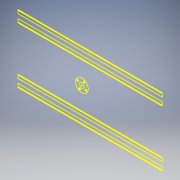
# Autodesk Inventor part: ZNutHolder
Saved by Autodesk Inventor 2019 (Build 230136000, 136)
## iProperties
Created: 2019-05-13
Part Number: ZNutHolder
Material: Generic
Document SubType Name: Modeling
Designer: Alex Jones
Density: 1 g/cm^3
Appearance: Default
Author: Alex Jones
Autodesk Inventor part; units mm, degrees
ref_plane "YZ Plane" through (0, 0, 0) normal (1, 0, 0) x (0, 1, 0)
ref_plane "XZ Plane" through (0, 0, 0) normal (0, 1, 0) x (-1, 0, 0)
ref_plane "XY Plane" through (0, 0, 0) normal (0, 0, 1) x (1, 0, 0)
sketch "Sketch1" plane through (0, 0, 0) normal (0, 0, 1) x (1, 0, 0)
  circle A0 centre (-131.3, 44.85) radius 1.5 projected
  circle A1 centre (-147.3, 44.85) radius 1.5 projected
  circle A2 centre (-139.3, 52.85) radius 1.5 projected
  circle A3 centre (-139.3, 36.85) radius 1.5 projected
  circle A4 centre (-139.3, 44.85) radius 4 projected
  circle A5 centre (-139.3, 44.85) radius 11 projected
  line L0 (-250, 102.05) -> (0, 102.05) projected
  line L1 (-250, 96.9) -> (-250, 102.05) projected
  line L2 (0, 96.9) -> (-250, 96.9) projected
  line L3 (0, 96.9) -> (0, 102.05) projected
  line L4 (0, 103.3) -> (-250, 103.3) projected
  line L5 (0, 84.55) -> (-250, 84.55) projected
  line L6 (0, 84.55) -> (0, 89.7) projected
  line L7 (0, 89.7) -> (-250, 89.7) projected
  line L8 (-250, 84.55) -> (-250, 89.7) projected
  line L9 (-250, 83.3) -> (0, 83.3) projected
  line L10 (-250, 5.15) -> (0, 5.15) projected
  line L11 (-250, 0) -> (-250, 5.15) projected
  line L12 (0, 0) -> (-250, 0) projected
  line L13 (0, 0) -> (0, 5.15) projected
  line L14 (0, -12.35) -> (-250, -12.35) projected
  line L15 (0, -12.35) -> (0, -7.2) projected
  line L16 (0, -7.2) -> (-250, -7.2) projected
  line L17 (-250, -12.35) -> (-250, -7.2) projected
  line L18 (-250, -13.6) -> (0, -13.6) projected
  line L19 (0, 6.4) -> (-250, 6.4) projected
  line L20 (-128.3, 103.3) -> (-150.3, 103.3)
  line L21 (-150.3, 103.3) -> (-150.3, -13.6)
  line L22 (-150.3, -13.6) -> (-128.3, -13.6)
  line L23 (-128.3, -13.6) -> (-128.3, 103.3)
  circle A6 centre (-139.3, 44.85) radius 5.5902
  constraints: 8 end point, 2 parallel, 2 point on line, 2 tangent, 1 centre point, 1 horizontal, 1 perpendicular
extrude "Extrusion1" add sketch "Sketch1" along normal blind 6.35 contours A5 | L23 L19 L21 A5 | A5 L21 L9 L23 | L23 L10 L21 L19 | L9 L21 L5 L23 | L23 L12 L21 L10 | L5 L21 L7 L23 | L23 L16 L21 L12 | L7 L21 L2 L23 | L23 L14 L21 L16 | L2 L21 L0 L23 | L23 L18 L21 L14 | L0 L21 L4 L23
sketch "Sketch2" plane through (0, 0, 0) normal (0, 0, -1) x (-1, 0, 0)
  line L0 (0, 5.15) -> (250, 5.15) projected
  line L1 (0, 5.15) -> (0, 0) projected
  line L2 (0, 0) -> (250, 0) projected
  line L3 (250, 5.15) -> (250, 0) projected
  line L4 (250, 6.4) -> (0, 6.4) projected
  line L5 (250, 84.55) -> (0, 84.55) projected
  line L6 (250, 89.7) -> (250, 84.55) projected
  line L7 (0, 89.7) -> (250, 89.7) projected
  line L8 (0, 89.7) -> (0, 84.55) projected
  line L9 (0, 83.3) -> (250, 83.3) projected
  circle A0 centre (139.3, 44.85) radius 5.5902 projected
  circle A1 centre (139.3, 36.85) radius 1.5 projected
  circle A2 centre (139.3, 52.85) radius 1.5 projected
  circle A3 centre (147.3, 44.85) radius 1.5 projected
  circle A4 centre (131.3, 44.85) radius 1.5 projected
  line L10 (128.3, 103.3) -> (150.3, 103.3) projected
  line L11 (128.3, -13.6) -> (128.3, 103.3) projected
  line L12 (150.3, -13.6) -> (128.3, -13.6) projected
  line L13 (150.3, 103.3) -> (150.3, -13.6) projected
  line L14 (128.3, -13.6) -> (128.3, 103.3) projected
  line L15 (150.3, 103.3) -> (150.3, -13.6) projected
  line L16 (128.3, 6.4) -> (150.3, 6.4)
  line L17 (150.3, 6.4) -> (150.3, 12.75)
  line L18 (150.3, 12.75) -> (128.3, 12.75)
  line L19 (128.3, 12.75) -> (128.3, 6.4)
  line L20 (128.3, 83.3) -> (150.3, 83.3)
  line L21 (150.3, 83.3) -> (150.3, 76.95)
  line L22 (150.3, 76.95) -> (128.3, 76.95)
  line L23 (128.3, 76.95) -> (128.3, 83.3)
  point P0 (0, 0)
  dimension "d2" = 6.35
  dimension "d3" = 6.35
  constraints: 16 end point, 6 point on line, 4 parallel, 2 horizontal, 2 perpendicular
  measures "d2" distance between parallel lines of L9 L22
  measures "d3" distance between parallel lines of L4 L18
ref_plane "Work Plane1" through (-250, -12.35, -20) normal (0, 0, -1) x (0, 1, 0)
extrude "Extrusion2" add sketch "Sketch2" along normal up to surface (20 mm away) contours L11 L18 L13 L4 | L11 L9 L13 L22
sketch "Sketch3" plane through (-128.3, -13.6, 6.35) normal (1, 0, 0) x (0, 0, -1)
  line L0 (6.35, 26.35) -> (26.35, 26.35) projected
  line L1 (26.35, 26.35) -> (6.35, 46.35)
  line L2 (6.35, 26.35) -> (6.35, 90.55) projected
  line L3 (6.35, 90.55) -> (26.35, 90.55) projected
  line L4 (26.35, 90.55) -> (6.35, 70.55)
  line L5 (6.35, 70.55) -> (6.35, 90.55)
  line L6 (26.35, 90.55) -> (6.35, 90.55)
  line L7 (6.35, 46.35) -> (6.35, 26.35)
  line L8 (26.35, 26.35) -> (6.35, 26.35)
  point P0 (6.35, 13.6)
  dimension "d6" = 45
  dimension "d7" = 45
  constraints: 12 end point, 2 collinear, 2 perpendicular, 2 point on line
  measures "d6" angle of L1 L2
  measures "d7" angle of L2 L4
extrude "Extrusion3" add sketch "Sketch3" against normal up to surface (22 mm away)
sketch "Sketch4" plane through (-128.3, 83.3, -20) normal (0, 0, -1) x (-1, 0, 0)
  line L0 (0, 0) -> (22, 0) projected
  line L1 (0, -6.35) -> (0, 0) projected
  line L2 (22, -6.35) -> (0, -6.35) projected
  line L3 (22, 0) -> (22, -6.35) projected
  line L4 (0, -76.9) -> (0, -70.55) projected
  line L5 (22, -76.9) -> (0, -76.9) projected
  line L6 (22, -70.55) -> (22, -76.9) projected
  line L7 (0, -70.55) -> (22, -70.55) projected
  line L8 (22, -26.35) -> (22, -6.35) projected
  line L9 (22, -6.35) -> (0, -6.35) projected
  line L10 (0, -26.35) -> (0, -6.35) projected
  line L11 (22, -26.35) -> (0, -26.35) projected
  line L12 (22, -70.55) -> (22, -50.55) projected
  line L13 (0, -50.55) -> (22, -50.55) projected
  line L14 (0, -70.55) -> (0, -50.55) projected
  line L15 (0, -70.55) -> (22, -70.55) projected
  line L16 (22, -6.35) -> (0, -6.35) projected
  line L17 (11, -6.35) -> (11, -70.55)
  line L18 (0, -70.55) -> (22, -70.55) projected
  line L19 (19.46, -70.55) -> (2.54, -70.55)
  line L20 (2.54, -70.55) -> (2.54, -6.35)
  line L21 (2.54, -6.35) -> (19.46, -6.35)
  line L22 (19.46, -6.35) -> (19.46, -70.55)
  line L23 (19.46, -70.55) -> (2.54, -6.35) construction
  line L24 (2.54, -70.55) -> (19.46, -6.35) construction
  point P0 (-128.3, -83.3)
  point P1 (11, -38.45)
  dimension "d10" = 2.54
  constraints: 14 end point, 5 midpoint, 2 parallel, 1 horizontal, 1 perpendicular, 1 point on line
  measures "d10" distance between parallel lines of L14 L20
extrude "Extrusion4" cut sketch "Sketch4" against normal up to surface (20 mm away) contours L2 L17 L11 L20 | L22 L11 L17 L2 | L11 L17 L13 L20 | L22 L13 L17 L11 | L13 L17 L7 L20 | L22 L7 L17 L13
sketch "Sketch5" plane through (-150.3, 6.4, 0) normal (0, -1, 0) x (1, 0, 0)
  line L0 (0, -20) -> (22, -20) projected
  line L1 (2.54, 0) -> (0, 0) projected
  line L2 (22, -20) -> (0, 0)
  circle A0 centre (11, -10) radius 2.75
  point P0 (150.3, 0)
  dimension "d13" = 5.5
  constraints: 2 end point, 1 centre point, 1 midpoint
  measures "d13" diameter of A0
extrude "Extrusion5" cut sketch "Sketch5" against normal through all
sketch "Sketch6" plane through (0, 0, 0) normal (0, 0, -1) x (-1, 0, 0)
  line L0 (128.3, 83.3) -> (150.3, 83.3) projected
  line L1 (128.3, 76.95) -> (128.3, 83.3) projected
  line L2 (130.84, 76.95) -> (128.3, 76.95) projected
  line L3 (147.76, 76.95) -> (130.84, 76.95) projected
  line L4 (150.3, 76.95) -> (147.76, 76.95) projected
  line L5 (150.3, 83.3) -> (150.3, 76.95) projected
  line L6 (128.3, 6.4) -> (128.3, 12.75) projected
  line L7 (150.3, 6.4) -> (128.3, 6.4) projected
  line L8 (150.3, 12.75) -> (150.3, 6.4) projected
  line L9 (147.76, 12.75) -> (150.3, 12.75) projected
  line L10 (130.84, 12.75) -> (147.76, 12.75) projected
  line L11 (128.3, 12.75) -> (130.84, 12.75) projected
  line L12 (128.3, 103.3) -> (150.3, 103.3) projected
  line L13 (150.3, -13.6) -> (128.3, -13.6) projected
  line L14 (139.3, 103.3) -> (139.3, 83.3)
  line L15 (139.3, 6.4) -> (139.3, -13.6)
  circle A0 centre (139.3, 93.3) radius 2.75
  circle A1 centre (139.3, -3.6) radius 2.75
  point P0 (0, 0)
  dimension "d16" = 5.5
  constraints: 6 midpoint, 4 end point, 2 centre point, 1 equal radius
  measures "d16" diameter of A0
extrude "Extrusion6" cut sketch "Sketch6" against normal through all contours A0 L14 | L14 A0 | A1 L15 | L15 A1
body "Solid1"
